Autodesk Inventor part; units mm, degrees
(part 2 of 2)
  line L956 (15.8214, 3.0524) -> (15.8318, 3.1132)
  line L957 (15.8318, 3.1132) -> (15.8442, 3.1734)
  line L958 (15.8442, 3.1734) -> (15.5913, 3.315)
  line L959 (15.5913, 3.315) -> (15.2554, 3.4241)
  line L960 (15.2554, 3.4241) -> (14.9676, 3.4583)
  line L961 (14.9676, 3.4583) -> (14.9422, 3.4023)
  line L962 (14.9422, 3.4023) -> (14.915, 3.3469)
  line L963 (14.915, 3.3469) -> (14.8562, 3.2378)
  line L964 (14.8562, 3.2378) -> (14.7929, 3.1303)
  line L965 (14.7929, 3.1303) -> (14.7259, 3.0241)
  line L966 (14.7259, 3.0241) -> (14.5818, 2.8156)
  line L967 (14.5818, 2.8156) -> (14.4261, 2.6115)
  line L968 (14.4261, 2.6115) -> (14.2601, 2.4115)
  line L969 (14.2601, 2.4115) -> (14.0847, 2.2154)
  line L970 (14.0847, 2.2154) -> (13.9004, 2.0233)
  line L971 (13.9004, 2.0233) -> (13.7077, 1.8349)
  line L972 (13.7077, 1.8349) -> (13.507, 1.6503)
  line L973 (13.507, 1.6503) -> (13.3514, 1.5144)
  line L974 (13.3514, 1.5144) -> (12.8549, 1.72)
  line L975 (12.8549, 1.72) -> (12.841, 1.9262)
  line L976 (12.841, 1.9262) -> (12.8296, 2.1986)
  line L977 (12.8296, 2.1986) -> (12.8265, 2.4681)
  line L978 (12.8265, 2.4681) -> (12.8321, 2.7343)
  line L979 (12.8321, 2.7343) -> (12.8466, 2.997)
  line L980 (12.8466, 2.997) -> (12.8707, 3.2557)
  line L981 (12.8707, 3.2557) -> (12.9049, 3.5101)
  line L982 (12.9049, 3.5101) -> (12.9505, 3.7595)
  line L983 (12.9505, 3.7595) -> (12.9781, 3.882)
  line L984 (12.9781, 3.882) -> (13.0095, 4.0027)
  line L985 (13.0095, 4.0027) -> (13.0451, 4.1215)
  line L986 (13.0451, 4.1215) -> (13.0649, 4.1799)
  line L987 (13.0649, 4.1799) -> (13.0865, 4.2374)
  line L988 (13.0865, 4.2374) -> (12.8589, 4.4167)
  line L989 (12.8589, 4.4167) -> (12.5442, 4.5771)
  line L990 (12.5442, 4.5771) -> (12.2654, 4.6558)
  line L991 (12.2654, 4.6558) -> (12.2315, 4.6045)
  line L992 (12.2315, 4.6045) -> (12.1959, 4.5541)
  line L993 (12.1959, 4.5541) -> (12.1208, 4.4555)
  line L994 (12.1208, 4.4555) -> (12.0415, 4.3592)
  line L995 (12.0415, 4.3592) -> (11.9586, 4.2649)
  line L996 (11.9586, 4.2649) -> (11.7837, 4.0814)
  line L997 (11.7837, 4.0814) -> (11.5981, 3.9042)
  line L998 (11.5981, 3.9042) -> (11.4028, 3.7326)
  line L999 (11.4028, 3.7326) -> (11.1989, 3.5664)
  line L1000 (11.1989, 3.5664) -> (10.9868, 3.4055)
  line L1001 (10.9868, 3.4055) -> (10.7669, 3.2496)
  line L1002 (10.7669, 3.2496) -> (10.5398, 3.0987)
  line L1003 (10.5398, 3.0987) -> (10.3649, 2.9888)
  line L1004 (10.3649, 2.9888) -> (9.9067, 3.2695)
  line L1005 (9.9067, 3.2695) -> (9.9252, 3.4753)
  line L1006 (9.9252, 3.4753) -> (9.9566, 3.7462)
  line L1007 (9.9566, 3.7462) -> (9.9957, 4.0128)
  line L1008 (9.9957, 4.0128) -> (10.0428, 4.2749)
  line L1009 (10.0428, 4.2749) -> (10.0983, 4.532)
  line L1010 (10.0983, 4.532) -> (10.1625, 4.7839)
  line L1011 (10.1625, 4.7839) -> (10.2362, 5.0298)
  line L1012 (10.2362, 5.0298) -> (10.3202, 5.2689)
  line L1013 (10.3202, 5.2689) -> (10.3666, 5.3856)
  line L1014 (10.3666, 5.3856) -> (10.4164, 5.5)
  line L1015 (10.4164, 5.5) -> (10.4702, 5.6116)
  line L1016 (10.4702, 5.6116) -> (10.499, 5.6662)
  line L1017 (10.499, 5.6662) -> (10.5293, 5.7197)
  line L1018 (10.5293, 5.7197) -> (10.3326, 5.9324)
  line L1019 (10.3326, 5.9324) -> (10.0468, 6.14)
  line L1020 (10.0468, 6.14) -> (9.7837, 6.2614)
  line L1021 (9.7837, 6.2614) -> (9.7422, 6.216)
  line L1022 (9.7422, 6.216) -> (9.6992, 6.1718)
  line L1023 (9.6992, 6.1718) -> (9.6096, 6.0862)
  line L1024 (9.6096, 6.0862) -> (9.5162, 6.0035)
  line L1025 (9.5162, 6.0035) -> (9.4196, 5.9233)
  line L1026 (9.4196, 5.9233) -> (9.2181, 5.7694)
  line L1027 (9.2181, 5.7694) -> (9.007, 5.6234)
  line L1028 (9.007, 5.6234) -> (8.7874, 5.4845)
  line L1029 (8.7874, 5.4845) -> (8.5599, 5.3523)
  line L1030 (8.5599, 5.3523) -> (8.3252, 5.2265)
  line L1031 (8.3252, 5.2265) -> (8.0837, 5.1069)
  line L1032 (8.0837, 5.1069) -> (7.8358, 4.9934)
  line L1033 (7.8358, 4.9934) -> (7.6459, 4.9122)
  line L1034 (7.6459, 4.9122) -> (7.2372, 5.2611)
  line L1035 (7.2372, 5.2611) -> (7.2877, 5.4615)
  line L1036 (7.2877, 5.4615) -> (7.361, 5.7241)
  line L1037 (7.361, 5.7241) -> (7.4414, 5.9813)
  line L1038 (7.4414, 5.9813) -> (7.5289, 6.2328)
  line L1039 (7.5289, 6.2328) -> (7.6239, 6.4781)
  line L1040 (7.6239, 6.4781) -> (7.7268, 6.7168)
  line L1041 (7.7268, 6.7168) -> (7.838, 6.9482)
  line L1042 (7.838, 6.9482) -> (7.9584, 7.1712)
  line L1043 (7.9584, 7.1712) -> (8.0225, 7.2792)
  line L1044 (8.0225, 7.2792) -> (8.0896, 7.3844)
  line L1045 (8.0896, 7.3844) -> (8.1602, 7.4863)
  line L1046 (8.1602, 7.4863) -> (8.1971, 7.5357)
  line L1047 (8.1971, 7.5357) -> (8.2354, 7.5837)
  line L1048 (8.2354, 7.5837) -> (8.0744, 7.8246)
  line L1049 (8.0744, 7.8246) -> (7.8246, 8.0744)
  line L1050 (7.8246, 8.0744) -> (7.5837, 8.2354)
  line L1051 (7.5837, 8.2354) -> (7.5357, 8.1971)
  line L1052 (7.5357, 8.1971) -> (7.4863, 8.1602)
  line L1053 (7.4863, 8.1602) -> (7.3844, 8.0896)
  line L1054 (7.3844, 8.0896) -> (7.2792, 8.0225)
  line L1055 (7.2792, 8.0225) -> (7.1712, 7.9584)
  line L1056 (7.1712, 7.9584) -> (6.9482, 7.838)
  line L1057 (6.9482, 7.838) -> (6.7168, 7.7268)
  line L1058 (6.7168, 7.7268) -> (6.4781, 7.6239)
  line L1059 (6.4781, 7.6239) -> (6.2328, 7.5289)
  line L1060 (6.2328, 7.5289) -> (5.9813, 7.4414)
  line L1061 (5.9813, 7.4414) -> (5.7241, 7.361)
  line L1062 (5.7241, 7.361) -> (5.4615, 7.2877)
  line L1063 (5.4615, 7.2877) -> (5.2611, 7.2372)
  line L1064 (5.2611, 7.2372) -> (4.9122, 7.6459)
  line L1065 (4.9122, 7.6459) -> (4.9934, 7.8358)
  line L1066 (4.9934, 7.8358) -> (5.1069, 8.0837)
  line L1067 (5.1069, 8.0837) -> (5.2265, 8.3252)
  line L1068 (5.2265, 8.3252) -> (5.3523, 8.5599)
  line L1069 (5.3523, 8.5599) -> (5.4845, 8.7874)
  line L1070 (5.4845, 8.7874) -> (5.6234, 9.007)
  line L1071 (5.6234, 9.007) -> (5.7694, 9.2181)
  line L1072 (5.7694, 9.2181) -> (5.9233, 9.4196)
  line L1073 (5.9233, 9.4196) -> (6.0035, 9.5162)
  line L1074 (6.0035, 9.5162) -> (6.0862, 9.6096)
  line L1075 (6.0862, 9.6096) -> (6.1718, 9.6992)
  line L1076 (6.1718, 9.6992) -> (6.216, 9.7422)
  line L1077 (6.216, 9.7422) -> (6.2614, 9.7837)
  line L1078 (6.2614, 9.7837) -> (6.14, 10.0468)
  line L1079 (6.14, 10.0468) -> (5.9324, 10.3326)
  line L1080 (5.9324, 10.3326) -> (5.7197, 10.5293)
  line L1081 (5.7197, 10.5293) -> (5.6662, 10.499)
  line L1082 (5.6662, 10.499) -> (5.6116, 10.4702)
  line L1083 (5.6116, 10.4702) -> (5.5, 10.4164)
  line L1084 (5.5, 10.4164) -> (5.3856, 10.3666)
  line L1085 (5.3856, 10.3666) -> (5.2689, 10.3202)
  line L1086 (5.2689, 10.3202) -> (5.0298, 10.2362)
  line L1087 (5.0298, 10.2362) -> (4.7839, 10.1625)
  line L1088 (4.7839, 10.1625) -> (4.532, 10.0983)
  line L1089 (4.532, 10.0983) -> (4.2749, 10.0428)
  line L1090 (4.2749, 10.0428) -> (4.0128, 9.9957)
  line L1091 (4.0128, 9.9957) -> (3.7462, 9.9566)
  line L1092 (3.7462, 9.9566) -> (3.4753, 9.9252)
  line L1093 (3.4753, 9.9252) -> (3.2695, 9.9067)
  line L1094 (3.2695, 9.9067) -> (2.9888, 10.3649)
  line L1095 (2.9888, 10.3649) -> (3.0987, 10.5398)
  line L1096 (3.0987, 10.5398) -> (3.2496, 10.7669)
  line L1097 (3.2496, 10.7669) -> (3.4055, 10.9868)
  line L1098 (3.4055, 10.9868) -> (3.5664, 11.1989)
  line L1099 (3.5664, 11.1989) -> (3.7326, 11.4028)
  line L1100 (3.7326, 11.4028) -> (3.9042, 11.5981)
  line L1101 (3.9042, 11.5981) -> (4.0814, 11.7837)
  line L1102 (4.0814, 11.7837) -> (4.2649, 11.9586)
  line L1103 (4.2649, 11.9586) -> (4.3592, 12.0415)
  line L1104 (4.3592, 12.0415) -> (4.4555, 12.1208)
  line L1105 (4.4555, 12.1208) -> (4.5541, 12.1959)
  line L1106 (4.5541, 12.1959) -> (4.6045, 12.2315)
  line L1107 (4.6045, 12.2315) -> (4.6558, 12.2654)
  line L1108 (4.6558, 12.2654) -> (4.5771, 12.5442)
  line L1109 (4.5771, 12.5442) -> (4.4167, 12.8589)
  line L1110 (4.4167, 12.8589) -> (4.2374, 13.0865)
  line L1111 (4.2374, 13.0865) -> (4.1799, 13.0649)
  line L1112 (4.1799, 13.0649) -> (4.1215, 13.0451)
  line L1113 (4.1215, 13.0451) -> (4.0027, 13.0095)
  line L1114 (4.0027, 13.0095) -> (3.882, 12.9781)
  line L1115 (3.882, 12.9781) -> (3.7595, 12.9505)
  line L1116 (3.7595, 12.9505) -> (3.5101, 12.9049)
  line L1117 (3.5101, 12.9049) -> (3.2557, 12.8707)
  line L1118 (3.2557, 12.8707) -> (2.997, 12.8466)
  line L1119 (2.997, 12.8466) -> (2.7343, 12.8321)
  line L1120 (2.7343, 12.8321) -> (2.4681, 12.8265)
  line L1121 (2.4681, 12.8265) -> (2.1986, 12.8296)
  line L1122 (2.1986, 12.8296) -> (1.9262, 12.841)
  line L1123 (1.9262, 12.841) -> (1.72, 12.8549)
  line L1124 (1.72, 12.8549) -> (1.5144, 13.3514)
  line L1125 (1.5144, 13.3514) -> (1.6503, 13.507)
  line L1126 (1.6503, 13.507) -> (1.8349, 13.7077)
  line L1127 (1.8349, 13.7077) -> (2.0233, 13.9004)
  line L1128 (2.0233, 13.9004) -> (2.2154, 14.0847)
  line L1129 (2.2154, 14.0847) -> (2.4115, 14.2601)
  line L1130 (2.4115, 14.2601) -> (2.6115, 14.4261)
  line L1131 (2.6115, 14.4261) -> (2.8156, 14.5818)
  line L1132 (2.8156, 14.5818) -> (3.0241, 14.7259)
  line L1133 (3.0241, 14.7259) -> (3.1303, 14.7929)
  line L1134 (3.1303, 14.7929) -> (3.2378, 14.8562)
  line L1135 (3.2378, 14.8562) -> (3.3469, 14.915)
  line L1136 (3.3469, 14.915) -> (3.4023, 14.9422)
  line L1137 (3.4023, 14.9422) -> (3.4583, 14.9676)
  line L1138 (3.4583, 14.9676) -> (3.4241, 15.2554)
  line L1139 (3.4241, 15.2554) -> (3.315, 15.5913)
  line L1140 (3.315, 15.5913) -> (3.1734, 15.8442)
  line L1141 (3.1734, 15.8442) -> (3.1132, 15.8318)
  line L1142 (3.1132, 15.8318) -> (3.0524, 15.8214)
  line L1143 (3.0524, 15.8214) -> (2.9296, 15.8047)
  line L1144 (2.9296, 15.8047) -> (2.8054, 15.7927)
  line L1145 (2.8054, 15.7927) -> (2.6801, 15.7846)
  line L1146 (2.6801, 15.7846) -> (2.4267, 15.7786)
  line L1147 (2.4267, 15.7786) -> (2.1701, 15.7845)
  line L1148 (2.1701, 15.7845) -> (1.9107, 15.8012)
  line L1149 (1.9107, 15.8012) -> (1.649, 15.828)
  line L1150 (1.649, 15.828) -> (1.3852, 15.8641)
  line L1151 (1.3852, 15.8641) -> (1.1195, 15.9093)
  line L1152 (1.1195, 15.9093) -> (0.8522, 15.9632)
  line L1153 (0.8522, 15.9632) -> (0.6508, 16.0092)
  line L1154 (0.6508, 16.0092) -> (0.5254, 16.5317)
  line L1155 (0.5254, 16.5317) -> (0.684, 16.6641)
  line L1156 (0.684, 16.6641) -> (0.8977, 16.8335)
  line L1157 (0.8977, 16.8335) -> (1.1139, 16.9944)
  line L1158 (1.1139, 16.9944) -> (1.3325, 17.1463)
  line L1159 (1.3325, 17.1463) -> (1.5536, 17.289)
  line L1160 (1.5536, 17.289) -> (1.777, 17.4216)
  line L1161 (1.777, 17.4216) -> (2.003, 17.5434)
  line L1162 (2.003, 17.5434) -> (2.2315, 17.6531)
  line L1163 (2.2315, 17.6531) -> (2.3469, 17.7028)
  line L1164 (2.3469, 17.7028) -> (2.463, 17.7484)
  line L1165 (2.463, 17.7484) -> (2.58, 17.7894)
  line L1166 (2.58, 17.7894) -> (2.6389, 17.8076)
  line L1167 (2.6389, 17.8076) -> (2.6981, 17.824)
  line L1168 (2.6981, 17.824) -> (2.7094, 18.1135)
  line L1169 (2.7094, 18.1135) -> (2.6542, 18.4624)
  line L1170 (2.6542, 18.4624) -> (2.554, 18.7343)
  line L1171 (2.554, 18.7343) -> (2.4925, 18.7315)
  line L1172 (2.4925, 18.7315) -> (2.4309, 18.7307)
  line L1173 (2.4309, 18.7307) -> (2.3069, 18.7335)
  line L1174 (2.3069, 18.7335) -> (2.1824, 18.741)
  line L1175 (2.1824, 18.741) -> (2.0574, 18.7526)
  line L1176 (2.0574, 18.7526) -> (1.8061, 18.7863)
  line L1177 (1.8061, 18.7863) -> (1.5536, 18.8323)
  line L1178 (1.5536, 18.8323) -> (1.3001, 18.8894)
  line L1179 (1.3001, 18.8894) -> (1.0457, 18.9568)
  line L1180 (1.0457, 18.9568) -> (0.7908, 19.0338)
  line L1181 (0.7908, 19.0338) -> (0.5355, 19.1199)
  line L1182 (0.5355, 19.1199) -> (0.2799, 19.215)
  line L1183 (0.2799, 19.215) -> (0.0882, 19.2919)
  line L1184 (0.0882, 19.2919) -> (0.046, 19.8276)
  line L1185 (0.046, 19.8276) -> (0.2234, 19.9336)
  line L1186 (0.2234, 19.9336) -> (0.461, 20.0674)
  line L1187 (0.461, 20.0674) -> (0.6996, 20.1925)
  line L1188 (0.6996, 20.1925) -> (0.9394, 20.3084)
  line L1189 (0.9394, 20.3084) -> (1.18, 20.4147)
  line L1190 (1.18, 20.4147) -> (1.4215, 20.5108)
  line L1191 (1.4215, 20.5108) -> (1.6637, 20.5957)
  line L1192 (1.6637, 20.5957) -> (1.9066, 20.6683)
  line L1193 (1.9066, 20.6683) -> (2.0283, 20.6993)
  line L1194 (2.0283, 20.6993) -> (2.1501, 20.7262)
  line L1195 (2.1501, 20.7262) -> (2.2721, 20.7484)
  line L1196 (2.2721, 20.7484) -> (2.3331, 20.7572)
  line L1197 (2.3331, 20.7572) -> (2.3942, 20.7641)
  line L1198 (2.3942, 20.7641) -> (2.4506, 21.0483)
  line L1199 (2.4506, 21.0483) -> (2.4506, 21.4015)
  circle A0 centre (21.2249, 21.2249) radius 0.5
  point P0 (0, 0)
  constraints: 2400 end point, 1 centre point
extrude "Extrusion7" add sketch "Sketch10" along normal blind 5
sketch "Sketch11" plane through (0, 5, 0) normal (0, 1, 0) x (1, 0, 0)
  circle A0 centre (-11.5469, -23.7422) radius 2.45 projected
  circle A1 centre (-30.9029, -18.7076) radius 2.45 projected
  arc A2 (-22.0443, -23.5325) -> (-21.6337, -23.6393) centre (-21.7856, -23.3806) ccw projected
  line L0 (-21.6337, -23.6393) -> (-18.9173, -22.0443) projected
  arc A3 (-18.9173, -22.0443) -> (-18.8105, -21.6337) centre (-19.0692, -21.7856) ccw projected
  line L1 (-18.8105, -21.6337) -> (-20.4055, -18.9173) projected
  arc A4 (-20.4055, -18.9173) -> (-20.8161, -18.8105) centre (-20.6642, -19.0692) ccw projected
  line L2 (-20.8161, -18.8105) -> (-23.5325, -20.4055) projected
  arc A5 (-23.5325, -20.4055) -> (-23.6393, -20.8161) centre (-23.3806, -20.6642) ccw projected
  line L3 (-23.6393, -20.8161) -> (-22.0443, -23.5325) projected
  circle A6 centre (-18.7076, -11.5469) radius 2.45 projected
  circle A7 centre (-23.7422, -30.9029) radius 2.45 projected
  circle A8 centre (-21.2249, -21.2249) radius 15 projected
  point P0 (0, 0)
extrude "Extrusion8" cut sketch "Sketch11" against normal up to next contours A0 | A1 | L3 A5 L2 A4 L1 A3 L0 A2 | A6 | A7
body "Solid3"
